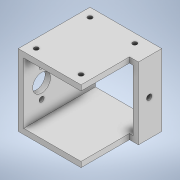
# Autodesk Inventor part: RD007
Saved by Autodesk Inventor 2021 (Build 250183000, 183)
## iProperties
Created: 2020-10-26
Part Number: RD007
Material: 一般
Document SubType Name: Modeling
Designer: ryusei
Density: 1 g/cm^3
Appearance: 既定
Author: ryusei
Title: ギアボックス(右)
Autodesk Inventor part; units mm, degrees
ref_plane "YZ Plane" through (0, 0, 0) normal (1, 0, 0) x (0, 1, 0)
ref_plane "XZ Plane" through (0, 0, 0) normal (0, 1, 0) x (-1, 0, 0)
ref_plane "XY Plane" through (0, 0, 0) normal (0, 0, 1) x (1, 0, 0)
sketch "スケッチ1" plane through (0, 0, 0) normal (0, 0, 1) x (1, 0, 0)
  line L0 (0, 0) -> (40, 0)
  line L1 (40, 0) -> (40, 40)
  line L2 (40, 40) -> (0, 40)
  line L3 (0, 40) -> (0, 0)
  line L4 (3, 37) -> (37, 37)
  line L5 (37, 37) -> (37, 3)
  line L6 (37, 3) -> (3, 3)
  line L7 (3, 3) -> (3, 37)
  dimension "d0" = 40
  dimension "d1" = 40
  dimension "d2" = 34
  constraints: 16 end point, 4 parallel, 2 perpendicular, 1 horizontal, 3 other
  measures "d0" distance between parallel lines of L1 L3
  measures "d1" distance between parallel lines of L0 L2
  measures "d2" distance between parallel lines of L5 L7
extrude "押し出し1" add sketch "スケッチ1" along normal blind 40
sketch "スケッチ2" plane through (40, 0, 0) normal (1, 0, 0) x (0, 0, -1)
  line L0 (-40, 40) -> (-13, 40)
  line L1 (-13, 40) -> (-13, 0)
  line L2 (-13, 0) -> (-40, 0)
  line L3 (-40, 0) -> (-40, 40)
  point P0 (0, 0)
  dimension "d5" = 27
  constraints: 8 end point, 2 parallel, 1 horizontal, 1 perpendicular
  measures "d5" distance between parallel lines of L1 L3
extrude "押し出し2" cut sketch "スケッチ2" against normal blind 5
sketch "スケッチ3" plane through (40, 0, 0) normal (1, 0, 0) x (0, 0, -1)
  line L0 (-13, 3) -> (-13, 37) projected
  line L1 (0, 37) -> (0, 3) projected
  line L2 (-40, 3) -> (-40, 37) construction
  line L3 (-13, 20) -> (0, 20) construction
  point P0 (0, 0)
  point P1 (-7, 20)
  dimension "d9" = 33
  constraints: 2 end point, 2 midpoint
  measures "d9" distance from line of L2 point (-7, 20)
hole "穴1" at (40, 20, 7) direction (-1, 0, 0) diameter 3 end through all
sketch "スケッチ5" plane through (0, 0, 0) normal (-1, 0, 0) x (0, 0, 1)
  line L0 (40, 40) -> (40, 0) projected
  line L1 (40, 20) -> (0, 20) construction
  line L2 (0, 3) -> (0, 37) projected
  point P0 (0, 0)
  point P1 (30, 20)
  dimension "d34" = 10
  constraints: 2 end point, 2 midpoint, 1 point on line
  measures "d34" distance from line of point (30, 20) L0
hole "穴3" at (0, 20, 30) direction (1, 0, 0) diameter 10 end through all
sketch "スケッチ6" plane through (0, 0, 0) normal (-1, 0, 0) x (0, 0, 1)
  line L0 (40, 3) -> (40, 37) projected
  line L1 (40, 20) -> (0, 20) construction
  line L2 (0, 3) -> (0, 37) projected
  line L3 (0, 0) -> (40, 0) projected
  point P0 (30, 12)
  point P1 (30, 28)
  dimension "d42" = 10
  dimension "d43" = 12
  constraints: 2 end point, 2 midpoint, 1 symmetric about line
  measures "d42" distance from line of point (30, 12) L0
  measures "d43" distance from line of point (30, 12) L3
hole "穴4" at (0, 12, 30) at (0, 28, 30) direction (1, 0, 0) diameter 2.8 end through all
sketch "スケッチ7" plane through (0, 40, 0) normal (0, 1, 0) x (1, 0, 0)
  line L0 (35, -40) -> (0, -40) projected
  line L1 (0, 0) -> (0, -40) projected
  point P0 (5, -35)
  point P1 (5, -5)
  point P2 (30, -35)
  point P3 (30, -5)
  dimension "d51" = 5
  dimension "d52" = 5
  dimension "d55" = 30
  dimension "d58" = 25
  constraints: 1 horizontal, 1 vertical, 3 other
  measures "d51" distance from line of L0 point (5, -35)
  measures "d52" distance from line of point (5, -35) L1
  measures "d55" distance of point (5, -35) point (5, -5)
  measures "d58" distance of point (5, -35) point (30, -35)
hole "穴5" at (5, 40, 35) at (5, 40, 5) at (30, 40, 35) at (30, 40, 5) direction (0, -1, 0) diameter 2.459 depth 3 tip angle 118 thread size "M3x0.5" class "6H" standard "ISO Metric profile"
